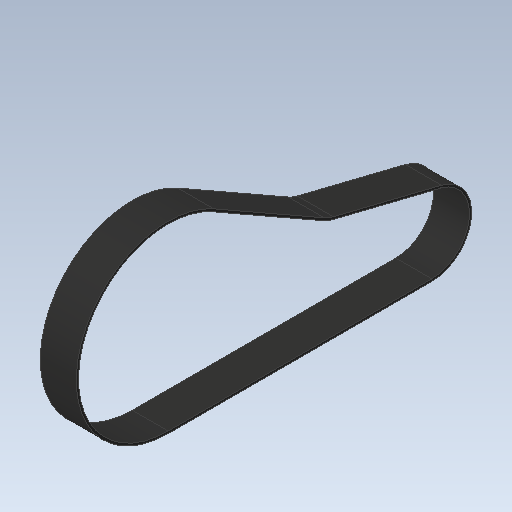
# Autodesk Inventor part: czesc2paska
Saved by Autodesk Inventor 2020 (Build 240168000, 168)
## iProperties
Created: 2020-08-27
Part Number: czesc2paska
Material: Rubber
Document SubType Name: Modeling
Designer: estee
Density: 0.93 g/cm^3
Appearance: Rubber - Black
Author: estee
Autodesk Inventor part; units mm, degrees
ref_plane "YZ Plane" through (0, 0, 0) normal (1, 0, 0) x (0, 1, 0)
ref_plane "XZ Plane" through (0, 0, 0) normal (0, 1, 0) x (-1, 0, 0)
ref_plane "XY Plane" through (0, 0, 0) normal (0, 0, 1) x (1, 0, 0)
sketch "Sketch1" plane through (0, 0, 0) normal (1, 0, 0) x (0, 1, 0)
  arc A0 (13.0108, -7.4161) -> (-14.976, 0) centre (0, 0) ccw
  arc A1 (-14.976, -44) -> (-2.6118, -45.5074) centre (-8.702, -44) ccw
  arc A2 (2.4963, -25.8629) -> (1.8506, -27.478) centre (8, -29) ccw
  line L0 (0, -65.4344) -> (0, 32.8066) projected
  line L1 (1.8506, -27.478) -> (-2.6118, -45.5074)
  line L2 (13.0108, -7.4161) -> (2.4963, -25.8629)
  line L3 (-14.976, 0) -> (-14.976, -44)
  arc A3 (13.3375, -7.6023) -> (-15.352, 0) centre (0, 0) ccw
  line L4 (13.3375, -7.6023) -> (2.8229, -26.0491)
  arc A4 (2.8229, -26.0491) -> (2.2155, -27.5683) centre (8, -29) ccw
  line L5 (2.2155, -27.5683) -> (-2.2468, -45.5977)
  arc A5 (-15.352, -44) -> (-2.2468, -45.5977) centre (-8.702, -44) ccw
  line L6 (-15.352, -44) -> (-15.352, 0)
  dimension "d0" = 29.952
  dimension "d1" = 12.548
  dimension "d2" = 12.67
  dimension "d3" = 29
  dimension "d4" = 44
  dimension "d5" = 8.702
  dimension "d6" = 8
  dimension "d7" = 0.376
  constraints: 12 end point, 12 point on circle, 6 centre point, 5 tangent, 1 coincident, 5 other
  measures "d0" diameter of A0
  measures "d1" diameter of A1
  measures "d2" diameter of A2
  measures "d3" vertical distance of A0.centre A2.centre
  measures "d4" vertical distance of A0.centre A1.centre
  measures "d5" distance from line of L0 A1.centre
  measures "d6" distance from line of L0 A2.centre
  measures "d7" radial gap between concentric circles of A0 A3
extrude "Extrusion1" add sketch "Sketch1" along normal mid plane 6 contours A0 L0 A3 L4 A4 L5 L1 A2 L2 | A0 L3 A1 L1 L0 L5 A5 L6 A3
body "Solid1"
